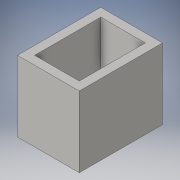
# Autodesk Inventor part: fc-GyroAccelBox
Saved by Autodesk Inventor 2016 SP1 (Build 200210100, 210)
## iProperties
Created: 2016-03-02
Part Number: fc-GyroAccelBox
Material: Generic
Document SubType Name: Modeling
Designer: steele
Density: 1 g/cm^3
Appearance: Default
Author: steele
Autodesk Inventor part; units mm, degrees
ref_plane "YZ Plane" through (0, 0, 0) normal (1, 0, 0) x (0, 1, 0)
ref_plane "XZ Plane" through (0, 0, 0) normal (0, 1, 0) x (-1, 0, 0)
ref_plane "XY Plane" through (0, 0, 0) normal (0, 0, 1) x (1, 0, 0)
sketch "Sketch1" plane through (0, 0, 0) normal (0, 1, 0) x (-1, 0, 0)
  line L0 (18.288, 24.638) -> (-18.288, 24.638)
  line L1 (-18.288, 24.638) -> (-18.288, -24.638)
  line L2 (-18.288, -24.638) -> (18.288, -24.638)
  line L3 (18.288, -24.638) -> (18.288, 24.638)
  line L4 (18.288, 24.638) -> (-18.288, -24.638) construction
  line L5 (-18.288, 24.638) -> (18.288, -24.638) construction
  point P0 (0, 0)
  dimension "d0" = 36.576
  dimension "d1" = 49.276
  constraints: 12 end point, 2 midpoint, 2 parallel, 1 horizontal, 1 perpendicular
  measures "d0" distance of L0.start L0.end
  measures "d1" distance of L2.end L0.start
extrude "Extrusion1" add sketch "Sketch1" along normal blind 41.91
sketch "Sketch3" plane through (0, 41.91, 0) normal (0, 1, 0) x (1, 0, 0)
  line L0 (-13.208, -19.558) -> (13.208, -19.558)
  line L1 (13.208, -19.558) -> (13.208, 19.558)
  line L2 (13.208, 19.558) -> (-13.208, 19.558)
  line L3 (-13.208, 19.558) -> (-13.208, -19.558)
  line L4 (-13.208, -19.558) -> (13.208, 19.558) construction
  line L5 (13.208, -19.558) -> (-13.208, 19.558) construction
  point P0 (0, 0)
  dimension "d4" = 26.416
  dimension "d5" = 39.116
  constraints: 12 end point, 2 midpoint, 2 parallel, 1 horizontal, 1 perpendicular
  measures "d4" distance of L0.start L0.end
  measures "d5" distance of L2.end L0.start
extrude "Extrusion2" cut sketch "Sketch3" against normal blind 36.83
equation "\"d0\" = 2 * printErrorThickness + boardWidth + 2 * boxWallThickness"
equation "\"d1\" = 2 * printErrorThickness + boardLength + 2 * boxWallThickness"
equation "\"d2\" = boxTotalHeight"
equation "\"d4\" = boardWidth + 2 * printErrorThickness"
equation "\"d5\" = boardLength + 2 * printErrorThickness"
equation "\"d6\" = interiorMaxHeight"
equation "\"boardWidth\" = 25.4"
equation "\"boardLength\" = 38.1"
equation "\"boardThickness\" = 5.08"
equation "\"boardLowerHeight\" = 5.08"
equation "\"boardUpperHeight\" = 6.35"
equation "\"boardHoleDiam\" = 2.286"
equation "\"boardHoleDistBetweenCenters\" = 19.05"
equation "\"boardHoleDistFromEnd\" = 5.08"
equation "\"boxBottomThickness\" = 5.08"
equation "\"boxWallThickness\" = 5.08"
equation "\"printErrorThickness\" = 0.508"
equation "\"boxTotalHeight\" = boardUpperHeight + boxBottomThickness + boardLowerHeight + boxClearance"
equation "\"boxClearance\" = 25.4"
equation "\"interiorMaxHeight\" = boxTotalHeight - boxBottomThickness"
body "Solid1"
